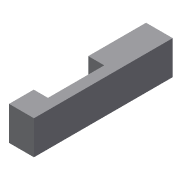
# Autodesk Inventor part: Claw base
Saved by Autodesk Inventor 2015 (Build 190159000, 159)
## iProperties
Created: 2015-02-09
Part Number: Claw base
Material: Generic
Document SubType Name: Modeling
Designer: Tanner
Density: 1 g/cm^3
Appearance: Default
Author: Tanner
Autodesk Inventor part; units mm, degrees
ref_plane "YZ Plane" through (0, 0, 0) normal (1, 0, 0) x (0, 1, 0)
ref_plane "XZ Plane" through (0, 0, 0) normal (0, 1, 0) x (-1, 0, 0)
ref_plane "XY Plane" through (0, 0, 0) normal (0, 0, 1) x (1, 0, 0)
sketch "Sketch1" plane through (0, 0, 0) normal (0, 0, 1) x (1, 0, 0)
  line L0 (0, 0) -> (19.05, 0)
  line L1 (19.05, 0) -> (19.05, 24.13)
  line L2 (19.05, 24.13) -> (0, 24.13)
  line L3 (0, 24.13) -> (0, 0)
  dimension "d0" = 19.05
  dimension "d1" = 24.13
  constraints: 8 end point, 2 parallel, 1 horizontal, 1 perpendicular
  measures "d0" distance of L2.end L1.end
  measures "d1" distance of L1.end L0.end
extrude "Extrusion1" add sketch "Sketch1" along normal blind 41.275
sketch "Sketch3" plane through (0, 0, 41.275) normal (0, 0, 1) x (1, 0, 0)
  line L0 (19.05, 24.13) -> (0, 24.13) projected
  line L1 (19.05, 0) -> (11.43, 0)
  line L2 (11.43, 0) -> (11.43, 24.13)
  line L3 (11.43, 24.13) -> (19.05, 24.13)
  line L4 (19.05, 24.13) -> (19.05, 0)
  line L5 (19.05, 0) -> (19.05, 24.13) projected
  point P0 (0, 0)
  dimension "d4" = 24.13
  dimension "d5" = 0
  dimension "d6" = 7.62
  constraints: 8 end point, 2 parallel, 1 horizontal, 1 perpendicular, 1 point on line
  measures "d4" distance of L3.end L1.start
  measures "d5" distance between parallel lines of L5 L4
  measures "d6" distance between parallel lines of L4 L2
extrude "Extrusion2" add sketch "Sketch3" along normal blind 57.8104
sketch "Sketch4" plane through (11.43, 0, 41.275) normal (-1, 0, 0) x (0, 0, 1)
  line L0 (-41.275, 24.13) -> (57.8104, 24.13) projected
  line L1 (57.8104, 0) -> (40.1828, 0)
  line L2 (40.1828, 0) -> (40.1828, 24.13)
  line L3 (40.1828, 24.13) -> (57.8104, 24.13)
  line L4 (57.8104, 24.13) -> (57.8104, 0)
  line L5 (57.8104, 24.13) -> (57.8104, 0) projected
  point P0 (-41.275, 0)
  dimension "d9" = 24.13
  dimension "d10" = 0
  dimension "d11" = 17.6276
  constraints: 8 end point, 2 parallel, 1 horizontal, 1 perpendicular, 1 point on line
  measures "d9" distance of L1.end L2.end
  measures "d10" distance between parallel lines of L4 L5
  measures "d11" distance between parallel lines of L2 L4
extrude "Extrusion3" add sketch "Sketch4" along normal blind 10.16
body "Solid1"
